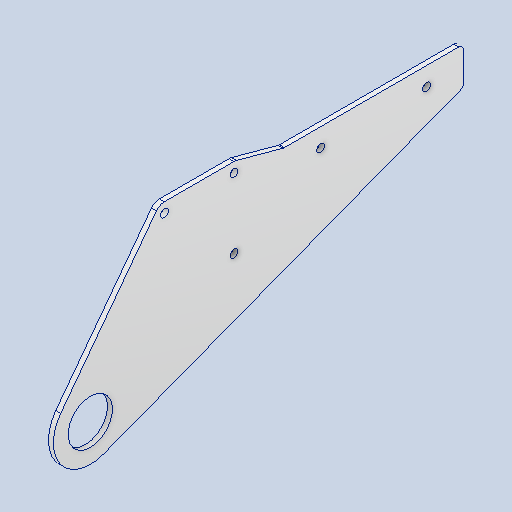
# Autodesk Inventor part: dribl-v3-Plate-3
Saved by Autodesk Inventor 2025.2 (Build 292293000, 293)
## iProperties
Created: 2025-04-04
Part Number: dribl-v3-Plate-3
Material: アルミニウム 6061
Document SubType Name: Modeling
Designer: haruy
Density: 2.7 g/cm^3
Appearance: アルミニウム - フラット
Author: haruy
Autodesk Inventor part; units mm, degrees
ref_plane "YZ Plane" through (0, 0, 0) normal (1, 0, 0) x (0, 1, 0)
ref_plane "XZ Plane" through (0, 0, 0) normal (0, 1, 0) x (-1, 0, 0)
ref_plane "XY Plane" through (0, 0, 0) normal (0, 0, 1) x (1, 0, 0)
derived "dribl-v3-Sketch-Base.ipt"
sketch "スケッチ1" plane through (400, 0, 0) normal (1, 0, 0) x (0, 1, 0)
  circle A0 centre (0, 0) radius 120 construction
  circle A1 centre (-96.5237, 35.1318) radius 6.5
  line L0 (0, 0) -> (-96.5237, 35.1318)
  line L1 (0, 0) -> (0, 120)
  line L2 (246.0862, 200) -> (-251.4603, 200)
  circle A2 centre (-67.6203, 200) radius 6.5
  line L3 (0, 0) -> (-120, 0)
  line L4 (248, 9.15) -> (186, 9.15)
  line L5 (186, 9.15) -> (186, -9.15)
  line L6 (186, -9.15) -> (248, -9.15)
  line L7 (248, -9.15) -> (248, 9.15)
  line L8 (186, 5.15) -> (178, 5.15)
  line L9 (178, 5.15) -> (178, -4.85)
  line L10 (178, -4.85) -> (186, -4.85)
  line L11 (186, -4.85) -> (186, 5.15)
  line L12 (178, 3.15) -> (173, 3.15)
  line L13 (173, 3.15) -> (173, -2.85)
  line L14 (173, -2.85) -> (178, -2.85)
  line L15 (178, -2.85) -> (178, 3.15)
  line L16 (173, 2.65) -> (158, 2.65)
  line L17 (158, 2.65) -> (158, -2.35)
  line L18 (158, -2.35) -> (173, -2.35)
  line L19 (173, -2.35) -> (173, 2.65)
  line L20 (186, 34.15) -> (184, 34.15)
  line L21 (184, 34.15) -> (184, -47.85)
  line L22 (184, -47.85) -> (186, -47.85)
  line L23 (186, -47.85) -> (186, 34.15)
  circle A3 centre (150, 65) radius 4
  circle A4 centre (150, 65) radius 14 construction
  line L24 (186, 34.15) -> (191, 34.15)
  line L25 (191, 34.15) -> (191, 14.15)
  line L26 (191, 14.15) -> (186, 14.15)
  line L27 (186, 14.15) -> (186, 34.15)
  line L28 (184, 34.15) -> (147.5804, 61.8148)
  line L29 (151.3835, 68.7531) -> (191, 54.15)
  line L30 (191, 54.15) -> (191, 34.15)
  line L31 (239.3868, 130) -> (-239.3868, 130)
  circle A5 centre (-96.5237, 35.1318) radius 4
  circle A6 centre (150, 65) radius 9
  line L32 (-92.7649, 33.7637) -> (-100.2825, 36.4998)
  line L33 (165, 36) -> (150, 36)
  circle A7 centre (150, 36) radius 5
  circle A8 centre (150, 36) radius 9
  circle A9 centre (-98.8174, 128.095) radius 6.5
  circle A10 centre (165, 36) radius 5
  line L34 (150, 65) -> (165, 36)
  circle A11 centre (165, 36) radius 9
  circle A12 centre (150, 65) radius 41.6497
  line L35 (150, 65) -> (150, 36)
  line L36 (150, 65) -> (-96.5237, 35.1318)
  line L37 (-98.8174, 128.095) -> (150, 65)
  line L38 (150, 65) -> (150, 23.3503)
  circle A13 centre (150, 65) radius 32.6497
  circle A14 centre (150, 32.3503) radius 9
  line L39 (166.9362, 23.3503) -> (134.8586, 23.3503)
  line L40 (174, 3.15) -> (174, -2.85)
  circle A15 centre (25, 0) radius 120
  line L41 (170, -52.2973) -> (211.3465, -67.3462)
  line L42 (211.3465, -67.3462) -> (205.1901, -84.2607)
  line L43 (205.1901, -84.2607) -> (163.8436, -69.2118)
  line L44 (163.8436, -69.2118) -> (170, -52.2973)
  line L45 (166.9218, -60.7546) -> (0, 0)
  line L46 (172.8191, -53.3234) -> (166.6627, -70.2379)
  line L47 (186, -47.85) -> (172.8191, -53.3234)
  line L48 (182.216, -56.7436) -> (176.0596, -73.6581)
  line L49 (186, -47.85) -> (191, -47.85)
  line L50 (191, -47.85) -> (191, -37.85)
  line L51 (191, -37.85) -> (186, -37.85)
  line L52 (186, -37.85) -> (186, -47.85)
  line L53 (191, -47.85) -> (182.216, -56.7436)
  circle A16 centre (221.5, -275) radius 6
  line L54 (211.5, 20) -> (208.5, 20)
  line L55 (208.5, 20) -> (208.5, -53.7075)
  line L56 (208.5, -53.7075) -> (211.5, -53.7075)
  line L57 (211.5, -53.7075) -> (211.5, 20)
  line L58 (211.5, 20) -> (231.5, 20)
  line L59 (231.5, 20) -> (231.5, -53.7075)
  line L60 (231.5, -53.7075) -> (211.5, -53.7075)
  line L61 (211.5, -53.7075) -> (211.5, 20)
  line L62 (-432.3334, -230) -> (-447.3334, -230) construction
  line L63 (-447.3334, -230) -> (-447.3334, -860) construction
  line L64 (-447.3334, -860) -> (-432.3334, -860) construction
  line L65 (-432.3334, -860) -> (-432.3334, -230) construction
  line L66 (-432.3334, -250) -> (-432.3334, -230) construction
  line L67 (343, -291.5) -> (278.5, -291.5)
  line L68 (278.5, -291.5) -> (278.5, -334.5)
  line L69 (278.5, -334.5) -> (343, -334.5)
  line L70 (343, -334.5) -> (343, -291.5)
  line L71 (278.5, -291.5) -> (293.5, -291.5)
  line L72 (293.5, -291.5) -> (293.5, -276.5)
  line L73 (293.5, -276.5) -> (278.5, -276.5)
  line L74 (278.5, -276.5) -> (278.5, -291.5)
  line L75 (211.5, -53.7075) -> (231.5, -53.7075)
  line L76 (231.5, -53.7075) -> (231.5, -305) construction
  line L77 (231.5, -305) -> (211.5, -305)
  line L78 (211.5, -305) -> (211.5, -53.7075) construction
  line L79 (-432.3334, -303) -> (-447.3334, -303)
  line L80 (-432.3334, -303) -> (875.6666, -303) construction
  line L81 (875.6666, -303) -> (875.6666, -323)
  line L82 (875.6666, -323) -> (-432.3334, -323) construction
  line L83 (-432.3334, -323) -> (-432.3334, -303)
  line L84 (278.5, -334.5) -> (293.5, -334.5)
  line L85 (293.5, -334.5) -> (293.5, -349.5)
  line L86 (293.5, -349.5) -> (278.5, -349.5)
  line L87 (278.5, -349.5) -> (278.5, -334.5)
  line L88 (278.5, -276.5) -> (263.5, -276.5)
  line L89 (263.5, -276.5) -> (263.5, -359.5)
  line L90 (263.5, -359.5) -> (278.5, -359.5)
  line L91 (278.5, -359.5) -> (278.5, -276.5)
  circle A17 centre (221.5, -275) radius 15 construction
  line L92 (231.5, -275) -> (211.5, -275)
  line L93 (211.5, -275) -> (211.5, -305)
  line L94 (211.5, -305) -> (231.5, -305)
  line L95 (231.5, -305) -> (231.5, -275)
  line L96 (226.5, -266.3397) -> (216.5, -283.6603)
  line L97 (242.4808, -298.6603) -> (252.4808, -281.3397) construction
  line L98 (216.5, -283.6603) -> (242.4808, -298.6603)
  line L99 (-524.3334, 10.1879) -> (-524.3334, -1075.6286) construction
  line L100 (278.5, -349.5) -> (263.5, -349.5)
  line L101 (278.5, -276.5) -> (225.8253, -260.6372) construction
  line L102 (263.5, -349.5) -> (209.9279, -284.544)
  line L103 (278.5, -313) -> (263.5, -313)
  circle A18 centre (271, -291.5) radius 1.6
  circle A19 centre (271, -334.5) radius 1.6
  circle A20 centre (221.5, -275) radius 9.1
  circle A21 centre (221.5, -275) radius 50 construction
  circle A22 centre (239.5, -334.8519) radius 12.5
  line L104 (221.5, -275) -> (237.3114, -322.4342)
  line L105 (221.5, -275) -> (178.1987, -300)
  line L106 (221.5, -275) -> (221.5, -225)
  line L107 (221.5, -275) -> (254.6735, -237.5899) construction
  circle A23 centre (259.5, -334.8519) radius 4 construction
  circle A24 centre (239.5, -354.8519) radius 4
  circle A25 centre (219.5, -334.8519) radius 4
  line L108 (206.6714, -277.2613) -> (215.5457, -335.4549)
  line L109 (216.6716, -337.6803) -> (236.6716, -357.6803)
  line L110 (263.5, -349.5) -> (240.9941, -358.5624)
  circle A26 centre (259.5, -334.8519) radius 1.6 construction
  circle A27 centre (239.5, -354.8519) radius 1.6
  circle A28 centre (219.5, -334.8519) radius 1.6
  line L111 (-452.3334, -283) -> (-432.3334, -283)
  line L112 (-432.3334, -283) -> (-432.3334, -663)
  line L113 (-432.3334, -663) -> (-452.3334, -663)
  line L114 (-452.3334, -663) -> (-452.3334, -283)
  line L115 (-464.8334, 407.9273) -> (-464.8334, -989.4099)
  line L116 (1035.1666, 407.9273) -> (1035.1666, -2194.3714)
  line L117 (-432.3334, -643) -> (-452.3334, -643)
  line L118 (-432.3334, -473) -> (-464.8334, -473)
  line L119 (-464.8334, -88) -> (1035.1666, -88)
  line L120 (1035.1666, 77) -> (-464.8334, 77)
  line L121 (875.6666, -303) -> (1005.1666, -303)
  line L122 (1005.1666, -303) -> (1005.1666, -323)
  line L123 (1005.1666, -323) -> (875.6666, -323)
  line L124 (875.6666, -323) -> (875.6666, -303)
  line L125 (1005.1666, -303) -> (980.1666, -303)
  line L126 (980.1666, -303) -> (980.1666, -323)
  line L127 (980.1666, -323) -> (1005.1666, -323)
  line L128 (1005.1666, -323) -> (1005.1666, -303)
  circle A29 centre (964.1666, -358.18) radius 16
  circle A30 centre (964.1666, -358.18) radius 7.5
  line L129 (976.8707, -387.2746) -> (-428.6466, -622.1068)
  line L130 (-428.6466, -622.1068) -> (-425.3507, -641.8333)
  line L131 (-425.3507, -641.8333) -> (980.1666, -407.0011)
  line L132 (980.1666, -407.0011) -> (976.8707, -387.2746)
  line L133 (-432.3334, -643) -> (-425.3507, -641.8333)
  line L134 (980.1666, -323) -> (980.1666, -407.0011)
  line L135 (-212.3334, -323) -> (-232.3334, -323)
  line L136 (-232.3334, -323) -> (-232.3334, -578)
  line L137 (-232.3334, -578) -> (-212.3334, -578)
  line L138 (-212.3334, -578) -> (-212.3334, -323)
  line L139 (-414.8334, 0) -> (-414.8334, -960.8427)
  line L140 (-432.3334, -323) -> (-432.3334, -622.7228)
  line L141 (-232.3334, 0) -> (-232.3334, -854.7037)
  line L142 (-232.3334, -303) -> (-127.3334, -303)
  line L143 (-127.3334, -303) -> (-127.3334, -379.18)
  line L144 (-127.3334, -379.18) -> (-232.3334, -379.18)
  line L145 (-232.3334, -379.18) -> (-232.3334, -303)
  line L146 (-164.3334, -303) -> (-184.3334, -303)
  line L147 (-184.3334, -303) -> (-184.3334, -323)
  line L148 (-184.3334, -323) -> (-164.3334, -323)
  line L149 (-164.3334, -323) -> (-164.3334, -303)
  line L150 (985.1666, -303) -> (985.1666, -323)
  circle A31 centre (-222.3334, -313) radius 1.6
  circle A32 centre (-202.3334, -313) radius 1.6
  circle A33 centre (-222.3334, -333) radius 1.6
  circle A34 centre (-222.3334, -353) radius 1.6
  circle A35 centre (-139.3334, -313) radius 1.6
  circle A36 centre (-149.3334, -313) radius 1.6
  circle A37 centre (-143.3334, -358.18) radius 16
  line L151 (948.1666, -303) -> (948.1666, -323)
  circle A38 centre (968.1666, -313) radius 1.5
  circle A39 centre (958.1666, -313) radius 1.5
  line L152 (957.1441, -390.5705) -> (960.44, -410.297)
  circle A40 centre (973.587, -397.9618) radius 1.5
  circle A41 centre (963.7237, -399.6098) radius 1.5
  line L153 (948.1666, -323) -> (948.1666, -358.18)
  line L154 (957.1441, -390.5705) -> (948.8361, -362.7598)
  circle A42 centre (221.5, -198) radius 15
  circle A43 centre (221.5, -198) radius 50 construction
  circle A44 centre (265.6942, -242.1942) radius 12.5 construction
  line L155 (221.5, -198) -> (265.6942, -242.1942)
  circle A45 centre (221.5, -198) radius 9
  circle A46 centre (265.6942, -242.1942) radius 20
  line L156 (265.6942, -242.1942) -> (279.8363, -256.3363)
  circle A47 centre (279.8363, -256.3363) radius 4
  circle A48 centre (279.8363, -256.3363) radius 1.6
  line L157 (279.8363, -228.052) -> (265.6942, -242.1942)
  line L158 (265.6942, -242.1942) -> (251.552, -256.3363)
  circle A49 centre (279.8363, -228.052) radius 4
  circle A50 centre (279.8363, -228.052) radius 1.6
  circle A51 centre (251.552, -256.3363) radius 4
  circle A52 centre (251.552, -256.3363) radius 1.6
  line L159 (230.5074, -186.0055) -> (282.2383, -224.8535)
  line L160 (-464.8334, -113) -> (1035.1666, -113)
  line L161 (283.8363, -228.052) -> (283.8363, -256.3363)
  line L162 (278.5, -276.5) -> (283.6962, -257.3856)
  line L163 (207.4935, -203.3681) -> (263.5, -349.5)
  line L164 (234.8545, -191.1694) -> (278.5, -276.5)
  circle A53 centre (265.6942, -242.1942) radius 6.6
  circle A54 centre (265.6942, -242.1942) radius 9.5
  circle A55 centre (272.4117, -248.9117) radius 1.6
  circle A56 centre (268.153, -233.0179) radius 1.6
  circle A57 centre (256.5179, -244.653) radius 1.6
  circle A58 centre (-422.3334, -313) radius 1.6
  circle A59 centre (-412.3334, -313) radius 1.6
  circle A60 centre (-402.3334, -313) radius 1.6
  circle A61 centre (-417.1354, -630.3221) radius 1.6
  circle A62 centre (-407.2721, -628.6742) radius 1.6
  circle A63 centre (-442.3334, -633) radius 1.6
  circle A64 centre (-442.3334, -623) radius 1.6
  line L165 (-452.3334, -613) -> (-432.3334, -613)
  line L166 (-399.0568, -617.1629) -> (-395.7609, -636.8895)
  line L167 (-428.6466, -622.1068) -> (-432.3334, -622.7228)
  line L168 (-232.3334, -193) -> (-212.3334, -193)
  line L169 (-212.3334, -193) -> (-212.3334, -753)
  line L170 (-212.3334, -753) -> (-232.3334, -753)
  line L171 (-232.3334, -753) -> (-232.3334, -193)
  line L172 (-212.3334, -443) -> (-192.3334, -443)
  line L173 (-192.3334, -443) -> (-192.3334, -463)
  line L174 (-192.3334, -463) -> (-212.3334, -463)
  line L175 (-212.3334, -463) -> (-212.3334, -443)
  line L176 (-212.3334, -593) -> (-192.3334, -593)
  line L177 (-192.3334, -593) -> (-192.3334, -613)
  line L178 (-192.3334, -613) -> (-212.3334, -613)
  line L179 (-212.3334, -613) -> (-212.3334, -593)
  line L180 (-212.3334, -638) -> (162.6666, -638)
  line L181 (162.6666, -638) -> (162.6666, -653)
  line L182 (162.6666, -653) -> (-212.3334, -653)
  line L183 (-212.3334, -653) -> (-212.3334, -638)
  line L184 (162.6666, -653) -> (177.6666, -653)
  line L185 (177.6666, -653) -> (177.6666, -668)
  line L186 (177.6666, -668) -> (162.6666, -668)
  line L187 (162.6666, -668) -> (162.6666, -653)
  line L188 (162.6666, -668) -> (147.6666, -668)
  line L189 (147.6666, -668) -> (147.6666, -524.7026)
  line L190 (147.6666, -524.7026) -> (162.6666, -524.7026)
  line L191 (162.6666, -524.7026) -> (162.6666, -668)
  circle A65 centre (155.1666, -534.7026) radius 1.6
  circle A66 centre (835.5011, -421.0331) radius 1.6
  circle A67 centre (855.2277, -417.7372) radius 1.6
  line L192 (235.1666, 77) -> (235.1666, -1482.2484)
  circle A68 centre (98.7026, -266.038) radius 120
  line L193 (865.1666, 77) -> (865.1666, -1796.5569)
  circle A69 centre (985.1666, 85) radius 120
  line L194 (98.7026, -266.038) -> (38.7026, -369.961)
  line L195 (98.7026, -266.038) -> (98.7026, -386.038)
  line L196 (98.7026, -266.038) -> (-17.2085, -297.0963)
  line L197 (98.7026, -266.038) -> (67.6443, -150.1269)
  line L198 (67.6443, -150.1269) -> (-17.2085, -297.0963)
  line L199 (98.7026, -266.038) -> (202.6256, -326.038)
  line L200 (100.0335, -128.2423) -> (277.6705, -230.8011)
  line L201 (170.0335, -6.9988) -> (347.6705, -109.5575)
  line L202 (1181.4736, 111) -> (1176.4736, 111)
  line L203 (1176.4736, 111) -> (1176.4736, 59)
  line L204 (1176.4736, 59) -> (1181.4736, 59)
  line L205 (1181.4736, 59) -> (1181.4736, 111)
  line L206 (1181.4736, 95) -> (1243.4736, 95)
  line L207 (1243.4736, 95) -> (1243.4736, 75)
  line L208 (1243.4736, 75) -> (1181.4736, 75)
  line L209 (1181.4736, 75) -> (1181.4736, 95)
  line L210 (1181.4736, 90) -> (1173.4736, 90)
  line L211 (1173.4736, 90) -> (1173.4736, 80)
  line L212 (1173.4736, 80) -> (1181.4736, 80)
  line L213 (1181.4736, 80) -> (1181.4736, 90)
  line L214 (1173.4736, 87.5) -> (1153.4736, 87.5)
  line L215 (1153.4736, 87.5) -> (1153.4736, 82.5)
  line L216 (1153.4736, 82.5) -> (1173.4736, 82.5)
  line L217 (1173.4736, 82.5) -> (1173.4736, 87.5)
  line L218 (1164.4736, 87.5) -> (1128.3456, 87.5)
  line L219 (1128.3456, 87.5) -> (1128.3456, 82.5)
  line L220 (1128.3456, 82.5) -> (1164.4736, 82.5)
  line L221 (1164.4736, 82.5) -> (1164.4736, 87.5)
  line L222 (1164.4736, 87.5) -> (1164.4736, 82.5)
  line L223 (1161.9856, 87.5) -> (1111.9856, 87.5)
  line L224 (1111.9856, 87.5) -> (1111.9856, 82.5)
  line L225 (1111.9856, 82.5) -> (1161.9856, 82.5)
  line L226 (1161.9856, 82.5) -> (1161.9856, 87.5)
  line L227 (1136.9856, 82.5) -> (1136.9856, 87.5)
  line L228 (1131.9856, 121) -> (1141.9856, 121)
  line L229 (1141.9856, 121) -> (1141.9856, 49)
  line L230 (1141.9856, 49) -> (1131.9856, 49)
  line L231 (1131.9856, 49) -> (1131.9856, 121)
  line L232 (1151.9856, 82.5) -> (1121.9856, 82.5)
  line L233 (1121.9856, 82.5) -> (1121.9856, 72.5)
  line L234 (1121.9856, 72.5) -> (1151.9856, 72.5)
  line L235 (1151.9856, 72.5) -> (1151.9856, 82.5)
  line L236 (1181.4736, 111) -> (1125.6464, 111)
  line L237 (1125.6464, 111) -> (1125.6464, 116)
  line L238 (1125.6464, 116) -> (1181.4736, 116)
  line L239 (1181.4736, 116) -> (1181.4736, 111)
  line L240 (1181.4736, 59) -> (1129.1207, 59)
  line L241 (1129.1207, 59) -> (1129.1207, 54)
  line L242 (1129.1207, 54) -> (1181.4736, 54)
  line L243 (1181.4736, 54) -> (1181.4736, 59)
  line L244 (1145.2356, 111) -> (1128.7356, 111)
  line L245 (1128.7356, 111) -> (1128.7356, 110)
  line L246 (1128.7356, 110) -> (1145.2356, 110)
  line L247 (1145.2356, 110) -> (1145.2356, 111)
  line L248 (1128.7356, 59) -> (1145.2356, 59)
  line L249 (1145.2356, 59) -> (1145.2356, 60)
  line L250 (1145.2356, 60) -> (1128.7356, 60)
  line L251 (1128.7356, 60) -> (1128.7356, 59)
  line L252 (1128.4856, 110) -> (1145.4856, 110)
  line L253 (1145.4856, 110) -> (1145.4856, 102.5)
  line L254 (1145.4856, 102.5) -> (1128.4856, 102.5)
  line L255 (1128.4856, 102.5) -> (1128.4856, 110)
  line L256 (1128.4856, 60) -> (1145.4856, 60)
  line L257 (1145.4856, 60) -> (1145.4856, 67.5)
  line L258 (1145.4856, 67.5) -> (1128.4856, 67.5)
  line L259 (1128.4856, 67.5) -> (1128.4856, 60)
  line L260 (1111.9856, 85) -> (1173.4736, 85)
  line L261 (129.8192, -150.1425) -> (13.8924, -350.9335)
  line L262 (1035.1666, 327) -> (-464.8334, 327)
  line L263 (928.1666, -303) -> (928.1666, -323)
  line L264 (913.1666, -276.5) -> (898.1666, -276.5)
  line L265 (898.1666, -276.5) -> (898.1666, -349.5)
  line L266 (898.1666, -349.5) -> (913.1666, -349.5)
  line L267 (913.1666, -349.5) -> (913.1666, -276.5)
  line L268 (913.1666, -276.5) -> (928.1666, -276.5)
  line L269 (928.1666, -276.5) -> (928.1666, -291.5)
  line L270 (928.1666, -291.5) -> (913.1666, -291.5)
  line L271 (913.1666, -291.5) -> (913.1666, -276.5)
  line L272 (913.1666, -349.5) -> (928.1666, -349.5)
  line L273 (928.1666, -349.5) -> (928.1666, -334.5)
  line L274 (928.1666, -334.5) -> (913.1666, -334.5)
  line L275 (913.1666, -334.5) -> (913.1666, -349.5)
  circle A70 centre (928.1666, -195) radius 52
  line L276 (928.1666, -291.5) -> (876.1666, -291.5)
  line L277 (876.1666, -291.5) -> (876.1666, -301.5)
  line L278 (876.1666, -301.5) -> (928.1666, -301.5)
  line L279 (928.1666, -301.5) -> (928.1666, -291.5)
  line L280 (1141.9856, 116) -> (1141.9856, 54)
  line L281 (899.9966, -209.3683) -> (1156.0139, 50.7856)
  line L282 (1156.0139, 50.7856) -> (1170.269, 36.7573)
  line L283 (1170.269, 36.7573) -> (914.2516, -223.3967)
  line L284 (914.2516, -223.3967) -> (899.9966, -209.3683)
  line L285 (1141.9856, 49) -> (1124.1397, 49)
  line L286 (1124.1397, 49) -> (1124.1397, 47)
  line L287 (1124.1397, 47) -> (1141.9856, 47)
  line L288 (1141.9856, 47) -> (1141.9856, 49)
  line L289 (1141.9856, 36.5306) -> (1156.2406, 22.5023)
  circle A71 centre (405.1666, 85) radius 120
  line L290 (285.1666, 327) -> (285.1666, -1249.7155)
  circle A72 centre (348.1666, -195) radius 52
  circle A73 centre (348.1666, -195) radius 285.7429
  point P0 (-60, 0)
  point P1 (875.6666, -313)
  point P2 (186, 0.15)
  point P3 (186, 0)
  point P4 (1136.9856, 49)
  dimension "d17" = 19
  dimension "d1" = 30
  dimension "d2" = 77
  dimension "d3" = 0
  dimension "d4" = 100
  dimension "d5" = 25
  dimension "d6" = 45
  dimension "d7" = 18
  dimension "d8" = 40
  dimension "d9" = 8
  dimension "d10" = 3.2
  dimension "d11" = 8
  dimension "d12" = 3.2
  dimension "d13" = 8
  dimension "d14" = 3.2
  dimension "d15" = 360
  dimension "d16" = 13.2
  dimension "d18" = 3.2
  dimension "d21" = 360
  measures "d1" diameter of A42
  measures "d2" distance of A42.centre point (221.5, -275)
  measures "d3" horizontal distance of point (221.5, -275) A42.centre
  measures "d4" diameter of A43
  measures "d5" diameter of A44
  measures "d7" diameter of A45
  measures "d8" diameter of A46
  measures "d9" diameter of A47
  measures "d10" diameter of A48
  measures "d11" diameter of A49
  measures "d12" diameter of A50
  measures "d13" diameter of A51
  measures "d14" diameter of A52
  measures "d15" distance between parallel lines of L118 L160
  measures "d16" diameter of A53
  measures "d18" diameter of A55
extrude "押し出し1" add sketch "スケッチ1" against normal blind 2 contours L192 L164 A42 L159 | L159 A49 A46 L200 L164 L192 | A42 L192 L200 A45 | A49 A46 A50 | L192 A42 L164 | L164 L200 L192 A42 | L161 A46 A47 L156 A55 A54 L157 A49 | A46 A49 L161 | L200 A45 L155 A42 | A49 L200 A46 | A46 A50 L157 L200 A49 | L200 A46 L164 | L164 A46 L155 L192 L200 | A42 L192 | A49 L157 A50 A46 | L161 A47 A46 | A42 L155 L192 L163 | L200 A49 L157 A54 A56 L155 L164 A46 | L200 L157 A49 | L164 L155 A46 | L200 A42 L192 | L192 L155 A42 L200 | A47 A46 A48 | A46 A48 L156 A47 | L74 L68 L103 L89 L88 | L164 A46 A47 L162 | L88 L89 L163 L192 L155 A46 A51 L164 | L155 A45 L200 A42 | L155 L164 A54 A57 L158 A51 A46 | L155 A54 L164 | L100 L89 L103 L68 L87 | A54 A55 L156 A53 L157 | L157 A53 L155 A54 A56 | A47 A46 L164 A54 A55 L156 | L156 A48 A46 A47 | A46 A51 L158 A54 L164 | A51 L158 A52 A46 | A46 A52 A51 | L155 A53 L164 A54 | L164 A53 L158 A54 A57 | A53 L156 L157 | L157 L155 A53 | A56 A54 | A54 A56 | A55 A54 L156 | L156 A54 A55 | A46 A52 L158 A51 | A54 L158 A53 L164 | L164 A53 L156 A55 A54 | L155 L158 L164 A53 | L164 L158 A53 | A57 A54 | A54 A57 | L156 A53 L164 L158 | A54 L156 A55 | A54 A55 L156 | A53 L158 L164
fillet "フィレット1" radius 2 3 edges at (399, 278.5, -276.5) (399, 278.5, -349.5) (399, 263.5, -349.5)
